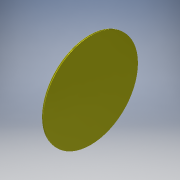
# Autodesk Inventor part: Pulley3d
Saved by Autodesk Inventor 2019 (Build 230136000, 136)
## iProperties
Created: 2017-01-18
Part Number: Pulley3d
Document SubType Name: Modeling
Designer: Administrator
Density: 1 g/cm^3
Mass: 2.38562 g
Surface Area: 27.2942 cm^2
Volume: 2.38562 cm^3
Material: Generic
Appearance: Smooth - Yellow
Author: Administrator
Autodesk Inventor part; units mm, degrees
ref_plane "YZ Plane" through (0, 0, 0) normal (1, 0, 0) x (0, 1, 0)
ref_plane "XZ Plane" through (0, 0, 0) normal (0, 1, 0) x (-1, 0, 0)
ref_plane "XY Plane" through (0, 0, 0) normal (0, 0, 1) x (1, 0, 0)
revolve "Revolution1" [suppressed]
sketch "Sketch2" plane through (0, 0, 0) normal (0, 0, 1) x (1, 0, 0)
  line L0 (0, -3) -> (0, 3) projected
  line L1 (0, 0) -> (-2.5, 0)
  line L2 (-2.5, 0) -> (-2.5, 90)
  line L3 (-2.5, 90) -> (0, 90) construction
  line L4 (0, 90) -> (0, 0)
  line L5 (-1.25, 90) -> (-1.25, 89) construction
  line L6 (-1.25, 89) -> (-1.7321, 89)
  line L7 (-1.7321, 89) -> (-2, 90)
  line L8 (-0.7679, 89) -> (-0.5, 90)
  line L9 (-0.7679, 89) -> (-1.25, 89)
  line L10 (-2, 90) -> (-2.5, 90)
  line L11 (-0.5, 90) -> (0, 90)
  dimension "d8" = 90
  dimension "d9" = 2.5
  dimension "d10" = 1
  dimension "d11" = 15
  dimension "d12" = 0.75
  constraints: 22 end point, 4 collinear, 3 perpendicular, 2 midpoint, 2 parallel, 2 symmetric about line, 1 point on line
  measures "d8" distance between parallel lines of L3 L1
  measures "d9" distance between parallel lines of L2 L4
  measures "d10" distance of L5.start L5.end
  measures "d11" angle of L7 L5
  measures "d12" distance from line of L5 L7.end
revolve "Revolution2" add sketch "Sketch2" angle 360 about axis through (0, 0, 0) along (-1, 0, 0)
sketch "Sketch3" plane through (16, 0, 0) normal (1, 0, 0) x (0, 0, -1)
  circle A0 centre (0, 0) radius 11 projected
  circle A1 centre (0, 0) radius 10 projected
  circle A2 centre (0, 0) radius 11 projected
  circle A3 centre (0, 7) radius 2.5
  circle A4 centre (0, 0) radius 3 construction
  dimension "d14" = 7
  dimension "d15" = 5
  dimension "d16" = 6
  constraints: 2 centre point, 1 coincident
  measures "d14" distance of A3.centre A0.centre
  measures "d15" diameter of A3
  measures "d16" diameter of A4
extrude "Extrusion1" [suppressed]
pattern_circular "Circular Pattern1" [suppressed]
sketch "Sketch4" plane through (16, 0, 0) normal (1, 0, 0) x (0, 0, -1)
  circle A0 centre (0, 0) radius 11 projected
  circle A1 centre (0, 0) radius 2.5
  dimension "d22" = 5
  constraints: 1 centre point, 1 coincident
  measures "d22" diameter of A1
extrude "Extrusion2" [suppressed]
body "Solid1"
